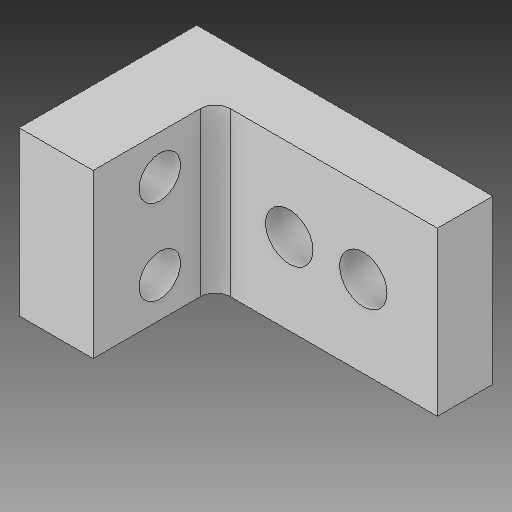
# Autodesk Inventor part: GlyphLiftHolder1
Saved by Autodesk Inventor 2019 (Build 230136000, 136)
## iProperties
Created: 2017-12-29
Part Number: GlyphLiftHolder1
Material: Generic
Document SubType Name: Modeling
Designer: Delta
Density: 1 g/cm^3
Appearance: Default
Author: Delta
Autodesk Inventor part; units mm, degrees
ref_plane "YZ Plane" through (0, 0, 0) normal (1, 0, 0) x (0, 1, 0)
ref_plane "XZ Plane" through (0, 0, 0) normal (0, 1, 0) x (-1, 0, 0)
ref_plane "XY Plane" through (0, 0, 0) normal (0, 0, 1) x (1, 0, 0)
sketch "Sketch1" plane through (0, 0, 0) normal (1, 0, 0) x (0, 1, 0)
  line L0 (0, 0) -> (13.97, 0)
  line L1 (13.97, 0) -> (13.97, -15.24)
  line L2 (13.97, -15.24) -> (0, -15.24)
  line L3 (0, -15.24) -> (0, 0)
  dimension "d0" = 13.97
  dimension "d1" = 15.24
  constraints: 8 end point, 2 parallel, 1 horizontal, 1 perpendicular
  measures "d0" distance of L1.end L2.end
  measures "d1" distance of L0.end L1.end
extrude "Extrusion1" add sketch "Sketch1" along normal blind 6.35
sketch "Sketch2" plane through (6.35, 0, 0) normal (1, 0, 0) x (0, 0, -1)
  line L0 (15.24, 0) -> (15.24, 13.97) projected
  line L1 (0, 0) -> (15.24, 0) projected
  line L2 (15.24, 13.97) -> (10.4775, 13.97)
  line L3 (10.4775, 13.97) -> (10.4775, 0)
  line L4 (10.4775, 0) -> (15.24, 0)
  line L5 (15.24, 0) -> (15.24, 13.97)
  dimension "d4" = 4.7625
  constraints: 8 end point, 2 parallel, 1 horizontal, 1 perpendicular, 1 point on line
  measures "d4" distance of L4.end L3.end
extrude "Extrusion2" add sketch "Sketch2" along normal blind 19.05
sketch "Sketch3" plane through (6.35, 0, 0) normal (1, 0, 0) x (0, 0, -1)
  line L0 (15.24, 0) -> (0, 0) projected
  line L1 (0, 0) -> (5.715, 0)
  line L2 (5.715, 0) -> (5.715, 3.3401)
  line L3 (0, 13.97) -> (15.24, 13.97) projected
  line L4 (5.715, 13.97) -> (5.715, 10.6299)
  line L5 (0, 13.97) -> (0, 0) projected
  line L6 (15.24, 0) -> (15.24, 13.97) projected
  dimension "d28" = 9.525
  dimension "d29" = 9.525
  dimension "d30" = 7.2898
  dimension "d31" = 3.3401
  dimension "d32" = 13.97
  constraints: 6 end point, 2 coincident, 2 point on line, 1 perpendicular, 1 vertical
  measures "d28" distance from line of L6 L4.end
  measures "d29" distance from line of L6 point (5.715, 3.34)
  measures "d30" distance of point (5.715, 3.34) L4.end
  measures "d31" distance from line of L0 point (5.715, 3.34)
  measures "d32" distance of L3.start L0.end
hole "Hole1" at (6.35, 10.6299, -5.715) at (6.35, 3.3401, -5.715) direction (-1, 0, 0) diameter 3.556 depth 25.4 tip angle 118
fillet "Fillet1" radius 1.27 1 edges at (6.35, 6.985, -10.4775)
sketch "Sketch4" plane through (25.4, 0, -10.4775) normal (0, 0, 1) x (1, 0, 0)
  line L0 (-17.78, 0) -> (0, 0) projected
  line L1 (0, 0) -> (0, 6.985)
  line L2 (0, 13.97) -> (0, 0) projected
  line L3 (0, 6.985) -> (-6.35, 6.985)
  line L4 (-19.05, 13.97) -> (-19.05, 0) projected
  line L5 (-19.05, 6.985) -> (-12.7, 6.985)
  point P0 (-25.4, 0)
  dimension "d19" = 6.35
  dimension "d20" = 6.35
  constraints: 6 end point, 2 coincident, 2 midpoint, 1 horizontal, 1 perpendicular
  measures "d19" distance of L1.end L3.end
  measures "d20" distance of L5.start L5.end
hole "Hole2" at (19.05, 6.985, -10.4775) at (12.7, 6.985, -10.4775) direction (0, 0, -1) diameter 4.064 depth 25.4 tip angle 118
equation "\"d29\" = d28"
equation "\"d31\" = -0.5 * d30 + 0.5 * d32"
body "Solid1"
